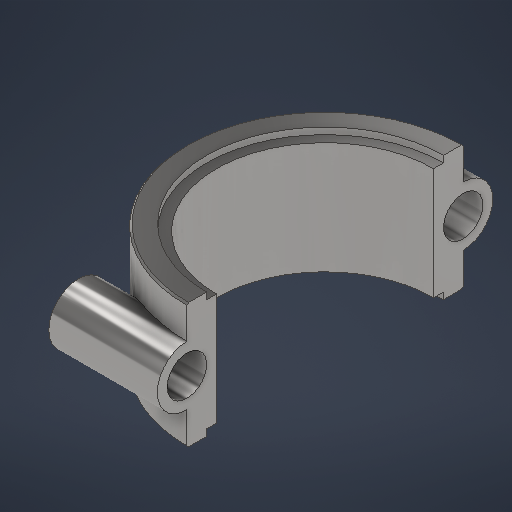
# Autodesk Inventor part: EM-004
Saved by Autodesk Inventor 2026.2 (Build 302298000, 298)
## iProperties
Company: CTE
Created: 2026-03-09
Part Number: EM-004
Material: Acero, alta resistencia, aleación baja
Document SubType Name: Modeling
Designer: Ing. Wilson Pinzón
Density: 7.85 g/cm^3
Appearance: Acero - Pulido
Mass: 346.496 g
Surface Area: 162.082 cm^2
Volume: 44.1396 cm^3
Author: Ing.Wilson Pinzón
Title: Acople de Biela
Autodesk Inventor part; units mm, degrees
ref_plane "YZ Plane" through (0, 0, 0) normal (1, 0, 0) x (0, 1, 0)
ref_plane "XZ Plane" through (0, 0, 0) normal (0, 1, 0) x (-1, 0, 0)
ref_plane "XY Plane" through (0, 0, 0) normal (0, 0, 1) x (1, 0, 0)
sketch "Boceto1" plane through (0, 0, 0) normal (0, 1, 0) x (-1, 0, 0)
  arc A0 (0, -33) -> (0, 33) centre (0, 0) ccw
  arc A1 (0, -36) -> (0, 36) centre (0, 0) ccw
  arc A2 (0, -42) -> (0, 42) centre (0, 0) ccw
  line L0 (0, -42) -> (0, 42)
  circle A3 centre (177, 0) radius 22
  circle A4 centre (177, 0) radius 18
  line L1 (159.2518, -13) -> (39.9375, -13)
  line L2 (159.2518, 13) -> (39.9375, 13)
  line L3 (139, 0) -> (57, 0) construction
  line L4 (139, 8) -> (57, 8)
  line L5 (57, -8) -> (139, -8)
  arc A5 (139, -8) -> (139, 8) centre (139, 0) ccw
  arc A6 (57, 8) -> (57, -8) centre (57, 0) ccw
  point P0 (98, 0)
  dimension "d0" = 66
  dimension "d1" = 72
  dimension "d2" = 84
  dimension "d3" = 44
  dimension "d4" = 177
  dimension "d5" = 36
  dimension "d6" = 26
  dimension "d7" = 41
  dimension "d8" = 16
  dimension "d9" = 57
  constraints: 14 end point, 14 point on circle, 7 centre point, 4 coincident, 4 point on line, 4 tangent, 2 horizontal, 2 horizontal alignment, 2 midpoint, 2 parallel, 2 vertical alignment, 1 vertical
  measures "d0" diameter of A0
  measures "d1" diameter of A1
  measures "d2" diameter of A2
  measures "d3" diameter of A3
  measures "d4" distance of point (0, 0) A3.centre
  measures "d5" diameter of A4
  measures "d6" distance between parallel lines of L2 L1
  measures "d7" distance of point (98, 0) L3.end
  measures "d8" diameter of A6
  measures "d9" distance of point (0, 0) L3.end
extrude "Extrusión1" add sketch "Boceto1" along normal mid plane 38 contours A1 L0 A2
extrude "Extrusión2" add sketch "Boceto1" along normal mid plane 34 contours A0 L0 A1
sketch "Boceto2" plane through (0, -19, -42) normal (1, 0, 0) x (0, 0, -1)
  line L0 (0, 0) -> (0, 38) projected
  circle A0 centre (0, 19) radius 9
  circle A1 centre (0, 19) radius 6
  point P0 (-42, 19)
  point P1 (0, 25)
  point P2 (0, 13)
  dimension "d18" = 18
  dimension "d19" = 12
  constraints: 2 centre point, 1 coincident, 1 midpoint
  measures "d18" diameter of A0
  measures "d19" diameter of A1
extrude "Extrusión5" cut sketch "Boceto2" against normal up to surface contours A1 L0 picked at (-1.87, 18.2908)
extrude "Extrusión6" add sketch "Boceto2" against normal blind 33 contours A0 L0 A1 | L0 A1 A0
mirror "Simetría1" about plane through (0, 0, 0) normal (0, 0, 1) of "Extrusión6", "Extrusión5"
chamfer "Chaflán2" distance 0.5 angle 45 2 edges at (-42, 19, 0) (-42, -19, 0)
